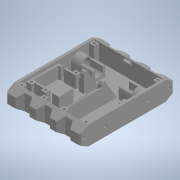
# Autodesk Inventor part: HexBodyV2
Saved by Autodesk Inventor 2020 (Build 240168000, 168)
## iProperties
Created: 2023-12-19
Part Number: HexBodyV2
Material: H TPU
Document SubType Name: Modeling
Designer: smz3rm
Density: 0.941117 g/cm^3
Appearance: Generic(1)
Mass: 179.09 g
Surface Area: 784.016 cm^2
Volume: 190.295 cm^3
BaseThickness: 3.000 mm
TopThickness: 1.778 mm
SideThickness: 4.000 mm
BodyWidth: 118.000 mm
BodyLength: 150.000 mm
BodyHeight: 30.000 mm
DriveMotorHeight: 15.000 mm
WheelWidth: 7.000 mm
WheelGrooveWidth: 5.000 mm
WheelGrooveDia: 18.000 mm
WheelDia: 45.000 mm
WheelPulleyDia: 2.500 mm
M3ScrewInsertBrim: 8.000 mm
M3ScrewDia: 3.100 mm
M3ScrewHeadDia: 6.100 mm
M3ScrewInsertDia: 4.000 mm
M3ScrewInsertDepth: 7.000 mm
DriveMotorOffset: 40.000 mm
DriveMotorHoleDia: 4.200 mm
M3ScrewHeadDepth: 2.200 mm
M3ScrewHeadTaper: -32.50 deg
WheeGuardlSlotWidth: 15.000 mm
WheelGuardScrewOffset: 7.000 mm
FlipperWidth: 20.000 mm
WheelSpokes: 5.000 ul
FlipperRodDia: 2.300 mm
FlipperArmThickness: 4.619 mm
FlipperArmLength: 87.010 mm
FlipperMountOffset: 70.000 mm
FlipperMountThickness: 6.000 mm
FlipperSpikeDrop: 40.009 mm
FlipperSpikeAngle: 30.00 deg
FlipperSpikeWidth: 10.000 mm
WheelGuardSpikeThickness: 8.000 mm
WheelGuardSpikeDrop: 37.700 mm
FlipperArmConnectorLength: 36.000 mm
VM3ScrewInsertDia: 3.750 mm
M2ScrewDia: 2.100 mm
WheelBearingDia: 7.150 mm
TopSupportWidth: 10.000 mm
TopSupportLength: 5.000 mm
ServoToFlipperAxisDistance: 13.685 mm
ServoHeightOffset: 3.000 mm
ServoGearCount: 15.000 ul
ServoGearCenterDistance: 21.290 mm
ServoGearRatio: 1.000 ul
ServoGearWidth: 10.000 mm
ServoToFlipperAxisAngle: 50.00 deg
RidgeCount: 4.000 ul
RidgeSpacing: 32.413 mm
RidgeLength: 20.762 mm
Author: smz3rm
Autodesk Inventor part; units mm, degrees
ref_plane "XZ Plane" through (0, 0, 0) normal (0, 1, 0) x (-1, 0, 0)
ref_plane "XY Plane" through (0, 0, 0) normal (0, 0, 1) x (1, 0, 0)
sketch "Sketch1" plane through (0, 0, 0) normal (1, 0, 0) x (0, 1, 0)
  line L0 (-15, 75) -> (15, 75)
  line L1 (15, 75) -> (15, -75)
  line L2 (15, -75) -> (-15, -75)
  line L3 (-15, -75) -> (-15, 75)
  line L4 (-15, 75) -> (15, -75) construction
  line L5 (15, 75) -> (-15, -75) construction
  line L6 (-21, 0) -> (21, 0) projected
  line L7 (0, -105) -> (0, 105) projected
  line L8 (7.5, -75) -> (-7.5, -75)
  line L9 (-7.5, -75) -> (-15, -62.0096)
  line L10 (-15, -62.0096) -> (-7.5, -49.0192)
  line L11 (-7.5, -49.0192) -> (7.5, -49.0192)
  line L12 (7.5, -49.0192) -> (15, -62.0096)
  line L13 (15, -62.0096) -> (7.5, -75)
  line L14 (-7.5, 75) -> (-15, 62.0096)
  line L15 (15, 62.0096) -> (7.5, 75)
  point P0 (0, 0)
  point P1 (0, -62.0096)
  point P2 (15, -62.0096)
  point P3 (15, 62.0096)
  point P4 (7.5, 75)
  point P5 (-7.5, 75)
  dimension "d0" = 30
  dimension "d1" = 150
  dimension "d25" = 12.9904
  constraints: 28 end point, 4 point on line, 4 symmetric about line, 2 midpoint, 2 parallel, 1 horizontal, 1 perpendicular, 13 other
  measures "d0" distance of L1.end L2.end
  measures "d1" distance of L0.end L1.end
  measures "d25" distance from line of point (0, -62.01) L2
extrude "Extrusion1" add sketch "Sketch1" along normal mid plane 118 contours L0 L7 L6 L3 L14 | L0 L15 L1 L6 L7 | L6 L7 L11 L10 L3 | L6 L1 L12 L11 L7 | L10 L11 L7 L2 L9 | L11 L12 L13 L2 L7
sketch "Sketch2" plane through (-59, 15, 62.4426) normal (0, 1, 0) x (1, 0, 0)
  line L0 (118, 124.4523) -> (118, 0.433) projected
  line L1 (0, 0.433) -> (0, 124.4523) projected
  line L2 (114, 124.4523) -> (4, 124.4523)
  line L3 (4, 124.4523) -> (4, 0.433)
  line L4 (4, 0.433) -> (114, 0.433)
  line L5 (114, 0.433) -> (114, 124.4523)
  line L6 (114, 124.4523) -> (4, 0.433) construction
  line L7 (4, 124.4523) -> (114, 0.433) construction
  line L8 (0, 0.433) -> (118, 0.433) projected
  line L9 (0, 124.4523) -> (118, 124.4523) projected
  line L10 (4, 124.0523) -> (114, 124.0523)
  line L11 (4, 0.833) -> (114, 0.833)
  point P0 (59, 62.4426)
  dimension "d4" = 4
  dimension "d89" = 0.4
  dimension "d90" = 0.4
  constraints: 16 end point, 5 point on line, 3 perpendicular, 2 midpoint, 2 parallel, 1 horizontal
  measures "d4" distance between parallel lines of L1 L3
  measures "d89" distance between parallel lines of L2 L10
  measures "d90" distance between parallel lines of L4 L11
extrude "Extrusion2" cut sketch "Sketch2" against normal blind 27 contours L5 L11 L3 L10
sketch "Sketch3" plane through (-59, -12, 62.4426) normal (0, 1, 0) x (1, 0, 0)
  line L0 (4, 0.833) -> (4, 124.0523) projected
  line L1 (114, 124.0523) -> (114, 0.833) projected
  line L2 (4, 0.833) -> (4, 124.0523) projected
  line L3 (114, 124.0523) -> (114, 0.833) projected
  line L4 (118, 124.4523) -> (118, 0.433) projected
  line L5 (0, 0.433) -> (0, 124.4523) projected
  line L6 (4, 124.0523) -> (12, 124.0523)
  line L7 (12, 124.0523) -> (12, 116.0523)
  line L8 (12, 116.0523) -> (4, 116.0523)
  line L9 (4, 116.0523) -> (4, 124.0523)
  line L10 (-23.6, 62.4426) -> (141.6, 62.4426) projected
  line L11 (59, 167.4426) -> (59, -42.5574) projected
  line L12 (106, 124.0523) -> (106, 116.0523)
  line L13 (106, 116.0523) -> (114, 116.0523)
  line L14 (12, 0.833) -> (12, 8.833)
  line L15 (12, 8.833) -> (4, 8.833)
  line L16 (106, 0.833) -> (106, 8.833)
  line L17 (106, 8.833) -> (114, 8.833)
  line L18 (0, 124.4523) -> (118, 124.4523) projected
  line L19 (0, 0.433) -> (118, 0.433) projected
  line L20 (114, 0.833) -> (4, 0.833) projected
  line L21 (4, 124.0523) -> (114, 124.0523) projected
  line L22 (114, 0.833) -> (4, 0.833) projected
  line L23 (4, 124.0523) -> (114, 124.0523) projected
  line L24 (4, 0.833) -> (4, 124.0523) projected
  line L25 (4, 124.0523) -> (114, 124.0523) projected
  point P0 (59, 62.4426)
  point P1 (4, 8.833)
  point P2 (4, 116.0523)
  point P3 (114, 116.0523)
  point P4 (114, 8.833)
  point P5 (12, 0.833)
  point P6 (106, 0.833)
  point P7 (12, 0.833)
  point P8 (106, 0.833)
  dimension "d8" = 8
  constraints: 20 end point, 9 symmetric about line, 2 horizontal, 2 parallel, 2 perpendicular, 1 collinear, 1 other
  measures "d8" distance of L7.end L8.end
extrude "Extrusion3" add sketch "Sketch3" along normal blind 25.222 contours L0 L15 L14 L20 | L0 L6 L7 L8 | L16 L17 L1 L20 | L13 L12 L21 L1
sketch "Sketch4" plane through (-55, 15, 62.0096) normal (1, 0, 0) x (0, 0, -1)
  circle A0 centre (97.0096, -15) radius 8.25
  line L0 (124.0192, -30) -> (0, -30) projected
  line L1 (137.0096, -7.5) -> (137.0096, -22.5) projected
  circle A1 centre (97.0096, -15) radius 10.25
  line L2 (86.7596, -15) -> (86.7596, -27)
  line L3 (8.4, -27) -> (115.6192, -27) projected
  line L4 (107.2596, -15) -> (107.2596, -27)
  point P0 (62.0096, -15)
  point P1 (0.4, -27)
  dimension "d12" = 16.5
  dimension "d13" = 15
  dimension "d14" = 40
  dimension "d15" = 2
  constraints: 4 end point, 2 centre point, 2 point on circle, 2 point on line, 2 tangent, 2 vertical, 1 coincident
  measures "d12" diameter of A0
  measures "d13" distance from line of L0 A0.centre
  measures "d14" distance from line of L1 A0.centre
  measures "d15" radial gap between concentric circles of A0 A1
extrude "Extrusion4" add sketch "Sketch4" along normal blind 14
sketch "Sketch5" plane through (-41, 15, 62.0096) normal (1, 0, 0) x (0, 0, -1)
  circle A0 centre (97.0096, -15) radius 8.25 projected
  circle A1 centre (97.0096, -15) radius 7.75
  arc A2 (107.2596, -15) -> (86.7596, -15) centre (97.0096, -15) ccw projected
  circle A3 centre (97.0096, -15) radius 8.25 projected
  line L0 (90.9096, -10.2196) -> (87.9426, -10.2196)
  arc A4 (107.2596, -15) -> (86.7596, -15) centre (97.0096, -15) ccw projected
  line L1 (90.9096, -10.2196) -> (90.9096, -27)
  line L2 (107.2596, -27) -> (86.7596, -27) projected
  line L3 (103.1096, -10.2196) -> (106.0766, -10.2196)
  line L4 (103.1096, -10.2196) -> (103.1096, -27)
  line L5 (86.7596, -15) -> (86.7596, -27) projected
  line L6 (107.2596, -27) -> (86.7596, -27) projected
  line L7 (107.2596, -27) -> (107.2596, -15) projected
  point P0 (62.0096, -15)
  point P1 (90.9096, -19.7804)
  point P2 (87.9426, -10.2196)
  point P3 (106.0766, -10.2196)
  point P4 (103.1096, -19.7804)
  dimension "d18" = 15.5
  dimension "d19" = 12.2
  constraints: 8 end point, 4 point on circle, 2 horizontal, 2 point on line, 1 centre point, 1 coincident, 1 parallel, 1 perpendicular
  measures "d18" diameter of A1
  measures "d19" distance between parallel lines of L4 L1
extrude "Extrusion5" add sketch "Sketch5" along normal blind 20 contours A0 L4 A1 L3 | A0 L3 A2 L7 L2 L4 | L4 L2 L1 A0 | A0 L1 A1 L4 | L0 A1 L1 A0 | A0 L1 L2 L5 A2 L0 | A1 L4 | L1 A1
sketch "Sketch6" plane through (-55, 0, -35) normal (1, 0, 0) x (0, 0, -1)
  circle A0 centre (0, 0) radius 2.1
  point P0 (-35, 0)
  dimension "d22" = 4.2
  constraints: 1 centre point
  measures "d22" diameter of A0
extrude "Extrusion6" cut sketch "Sketch6" against normal through all
mirror "Mirror1" about plane through (0, 0, 0) normal (1, 0, 0) of "Extrusion4", "Extrusion5", "Extrusion6"
sketch "Sketch7" plane through (-59, 0, 0) normal (-1, 0, 0) x (0, 0, 1)
  line L0 (-105, 0) -> (105, 0) projected
  circle A0 centre (35, 0) radius 2
  line L1 (75, -7.5) -> (75, 7.5) projected
  point P0 (0, 0)
  dimension "d26" = 4
  dimension "d27" = 40
  constraints: 1 centre point, 1 point on line
  measures "d26" diameter of A0
  measures "d27" distance from line of L1 A0.centre
extrude "Extrusion7" cut sketch "Sketch7" against normal up to surface (4 mm away)
mirror "Mirror2" about plane through (0, 0, 0) normal (1, 0, 0) of "Extrusion7"
sketch "Sketch9" plane through (-59, 0, 0) normal (-1, 0, 0) x (0, 0, 1)
  line L0 (-75, -7.5) -> (-75, 7.5) projected
  line L1 (-75, 0) -> (-62.0096, 0)
  circle A0 centre (-68.5048, 0) radius 2
  line L2 (0, -21) -> (0, 21) projected
  circle A1 centre (68.5048, 0) radius 2
  line L3 (-75, -7.5) -> (-62.0096, -15) projected
  line L4 (-62.0096, -15) -> (-62.0096, 15)
  point P0 (0, 0)
  dimension "d30" = 4
  constraints: 4 end point, 4 midpoint, 2 centre point, 1 symmetric about line, 1 vertical, 1 other
  measures "d30" diameter of A0
extrude "Extrusion8" cut sketch "Sketch9" against normal blind 7 contours A0 L1 | L1 A0 | A1
mirror "Mirror3" about plane through (0, 0, 0) normal (1, 0, 0) of "Extrusion8"
ref_plane "Work Plane1" through (11, 0, 0) normal (1, 0, 0) x (0, 1, 0)
sketch "Sketch10" plane through (11, 0, 0) normal (1, 0, 0) x (0, 1, 0)
  line L0 (-12, 61.6096) -> (-12, -24.75) projected
  line L1 (-12, -1.3627) -> (20.4594, -1.3627)
  line L2 (20.4594, -1.3627) -> (20.4594, -6.8187)
  line L3 (20.4594, -6.8187) -> (-12, -25.5591)
  circle A0 centre (17.3094, -5) radius 1.15
  line L4 (-7.5, -75) -> (7.5, -75) projected
  line L5 (15, -62.0096) -> (15, 62.0096) projected
  line L6 (-12, -24.75) -> (-12, -45.25) projected
  line L7 (-12, -61.6096) -> (-12, 53.6096) projected
  line L8 (20.4594, -6.8187) -> (17.3094, -8.6373)
  line L9 (17.3094, -8.6373) -> (14.1594, -6.8187)
  line L10 (14.1594, -6.8187) -> (14.1594, -3.1813)
  line L11 (14.1594, -3.1813) -> (17.3094, -1.3627)
  line L12 (17.3094, -1.3627) -> (20.4594, -3.1813)
  line L13 (20.4594, -3.1813) -> (20.4594, -6.8187)
  point P0 (0, 0)
  point P1 (18.4594, -5)
  point P2 (15, -9.9706)
  point P3 (15, -1.3627)
  point P4 (-12, -53.6096)
  point P5 (-12, 53.6096)
  dimension "d34" = 2.3
  dimension "d38" = 70
  dimension "d40" = 1.15
  dimension "d41" = 2.3094
  dimension "d44" = 60
  dimension "d45" = 2
  constraints: 18 end point, 4 point on line, 1 coincident, 1 collinear, 1 horizontal, 1 horizontal alignment, 1 perpendicular, 15 other
  measures "d38" distance from line of L4 point (17.309, -5)
  measures "d40" distance of point (17.309, -5) point (18.459, -5)
  measures "d41" distance from line of L5 point (17.309, -5)
  measures "d44" angle of L0 L3
  measures "d45" distance from line of L13 point (18.459, -5)
extrude "Extrusion9" add sketch "Sketch10" along normal blind 6 contours L1 L5 L11 L10 L9 L3 L6 L0 | L1 L11 L5 | L12 L2 L3 L9 L5 L11 | L5 L9 L10 L11 | L5 L9 L3
mirror "Mirror4" about plane through (0, 0, 0) normal (1, 0, 0) of "Extrusion9"
sketch "Sketch12" plane through (-59, -12, 62.4426) normal (0, 1, 0) x (1, 0, 0)
  line L0 (114, 116.0523) -> (114, 107.6926) projected
  line L1 (114, 116.0523) -> (106, 116.0523) projected
  line L2 (106, 116.0523) -> (106, 124.0523) projected
  line L3 (12, 124.0523) -> (12, 116.0523) projected
  line L4 (12, 116.0523) -> (4, 116.0523) projected
  line L5 (4, 107.6926) -> (4, 116.0523) projected
  line L6 (4, 8.833) -> (12, 8.833) projected
  line L7 (12, 8.833) -> (12, 0.833) projected
  line L8 (106, 0.833) -> (106, 8.833) projected
  line L9 (106, 8.833) -> (114, 8.833) projected
  line L10 (47, 0.833) -> (39, 0.833)
  line L11 (39, 0.833) -> (39, 8.833)
  line L12 (39, 8.833) -> (47, 8.833)
  line L13 (47, 8.833) -> (47, 0.833)
  line L14 (59, 167.4426) -> (59, -42.5574) projected
  line L15 (79, 0.833) -> (79, 8.833)
  line L16 (79, 8.833) -> (71, 8.833)
  line L17 (71, 8.833) -> (71, 0.833)
  line L18 (12, 124.0523) -> (106, 124.0523) projected
  line L19 (106, 0.833) -> (12, 0.833) projected
  line L20 (114, 87.1926) -> (80, 87.1926) projected
  line L21 (80, 87.1926) -> (80, 107.6926) projected
  line L22 (80, 107.6926) -> (114, 107.6926) projected
  line L23 (4, 107.6926) -> (38, 107.6926) projected
  line L24 (38, 107.6926) -> (38, 87.1926) projected
  line L25 (38, 87.1926) -> (4, 87.1926) projected
  line L26 (4, 8.833) -> (4, 87.1926) projected
  line L27 (114, 87.1926) -> (114, 8.833) projected
  line L28 (76, 63.8053) -> (70, 63.8053) projected
  line L29 (48, 63.8053) -> (42, 63.8053) projected
  line L30 (70, 63.8053) -> (76, 63.8053) projected
  line L31 (48, 63.8053) -> (42, 63.8053) projected
  line L32 (42, 88.0017) -> (48, 88.0017) projected
  line L33 (48, 88.0017) -> (48, 63.8053) projected
  line L34 (48, 63.8053) -> (42, 63.8053) projected
  line L35 (42, 63.8053) -> (42, 88.0017) projected
  line L36 (76, 88.0017) -> (76, 63.8053) projected
  line L37 (76, 63.8053) -> (70, 63.8053) projected
  line L38 (70, 63.8053) -> (70, 88.0017) projected
  line L39 (70, 88.0017) -> (76, 88.0017) projected
  point P0 (59, 62.4426)
  point P1 (71, 0.833)
  point P2 (79, 0.833)
  dimension "d46" = 8
  dimension "d55" = 12
  constraints: 14 end point, 4 symmetric about line, 2 parallel, 2 perpendicular, 1 collinear, 1 horizontal
  measures "d46" distance of L11.end L12.end
  measures "d55" distance between parallel lines of L14 L13
extrude "Extrusion10" add sketch "Sketch12" along normal blind 25.222 contours L17 L16 L15 L19 | L10 L11 L12 L13
sketch "Sketch13" plane through (-59, 13.222, 62.4426) normal (0, 1, 0) x (1, 0, 0)
  line L0 (12, 116.0523) -> (12, 124.0523) projected
  line L1 (4, 124.0523) -> (12, 124.0523) projected
  line L2 (4, 116.0523) -> (4, 124.0523) projected
  line L3 (4, 116.0523) -> (12, 116.0523) projected
  line L4 (106, 124.0523) -> (114, 124.0523) projected
  line L5 (106, 124.0523) -> (106, 116.0523) projected
  line L6 (106, 116.0523) -> (114, 116.0523) projected
  line L7 (114, 124.0523) -> (114, 116.0523) projected
  line L8 (12, 0.833) -> (4, 0.833) projected
  line L9 (12, 0.833) -> (12, 8.833) projected
  line L10 (12, 8.833) -> (4, 8.833) projected
  line L11 (4, 0.833) -> (4, 8.833) projected
  line L12 (47, 0.833) -> (39, 0.833) projected
  line L13 (47, 0.833) -> (47, 8.833) projected
  line L14 (47, 8.833) -> (39, 8.833) projected
  line L15 (39, 8.833) -> (39, 0.833) projected
  line L16 (114, 8.833) -> (114, 0.833) projected
  line L17 (114, 8.833) -> (106, 8.833) projected
  line L18 (106, 8.833) -> (106, 0.833) projected
  line L19 (114, 0.833) -> (106, 0.833) projected
  line L20 (79, 0.833) -> (79, 8.833) projected
  line L21 (79, 8.833) -> (71, 8.833) projected
  line L22 (71, 8.833) -> (71, 0.833) projected
  line L23 (79, 0.833) -> (71, 0.833) projected
  circle A0 centre (8, 120.0523) radius 1.875
  line L24 (4, 116.0523) -> (4, 124.0523) projected
  line L25 (4, 120.0523) -> (12, 120.0523)
  line L26 (4, 124.0523) -> (12, 124.0523) projected
  line L27 (8, 124.0523) -> (8, 116.0523)
  line L28 (12, 116.0523) -> (4, 116.0523) projected
  line L29 (-23.6, 62.4426) -> (141.6, 62.4426) projected
  line L30 (59, 167.4426) -> (59, -42.5574) projected
  circle A1 centre (110, 120.0523) radius 1.875
  circle A2 centre (8, 4.833) radius 1.875
  circle A3 centre (110, 4.833) radius 1.875
  circle A4 centre (43, 4.833) radius 1.875
  line L31 (39, 0.833) -> (39, 8.833) projected
  line L32 (39, 4.833) -> (47, 4.833)
  line L33 (47, 8.833) -> (39, 8.833) projected
  line L34 (43, 8.833) -> (43, 0.833)
  circle A5 centre (75, 4.833) radius 1.875
  dimension "d91" = 3.75
  dimension "d92" = 3.75
  constraints: 10 midpoint, 8 end point, 6 centre point, 4 symmetric about line, 4 other
  measures "d91" diameter of A0
  measures "d92" diameter of A4
extrude "Extrusion11" cut sketch "Sketch13" against normal blind 7 contours L25 L27 A0 | A0 L27 L25 | A0 L25 L27 | L27 L25 A0 | L34 L32 A4 | A4 L32 L34 | L32 L34 A4 | A4 L34 L32 | A1 | A2 | A3 | A5
sketch "Sketch14" plane through (-59, -12, 62.4426) normal (0, 1, 0) x (1, 0, 0)
  line L0 (7, 63.7574) -> (48, 63.7574)
  line L1 (48, 63.7574) -> (48, 23.7574)
  line L2 (48, 23.7574) -> (7, 23.7574)
  line L3 (7, 23.7574) -> (7, 63.7574)
  line L4 (51, 66.7574) -> (4.5, 66.7574)
  line L5 (4.5, 20.7574) -> (51, 20.7574)
  line L6 (51, 20.7574) -> (51, 66.7574)
  line L7 (40, 66.7574) -> (40, 20.7574)
  line L8 (35, 66.7574) -> (35, 20.7574)
  line L9 (7, 63.7574) -> (35, 63.7574)
  line L10 (4, 43.7574) -> (51, 43.7574)
  line L11 (15.5, 66.7574) -> (15.5, 63.7574)
  line L12 (11, 66.7574) -> (11, 63.7574)
  line L13 (48, 53.7574) -> (54, 53.7574)
  line L14 (54, 53.7574) -> (59, 53.7574)
  line L15 (59, 167.4426) -> (59, -42.5574) projected
  line L16 (48, 68.5926) -> (48, 66.2926) projected
  line L17 (4.5, 66.7574) -> (4, 66.7574)
  line L18 (4, 8.833) -> (4, 87.1926) projected
  line L19 (4, 0.833) -> (4, 124.0523) projected
  line L20 (4.5, 20.7574) -> (4, 20.7574)
  line L21 (35, 23.7574) -> (27, 23.7574)
  line L22 (27, 23.7574) -> (27, 15.7574)
  line L23 (27, 15.7574) -> (35, 15.7574)
  line L24 (35, 15.7574) -> (35, 23.7574)
  line L25 (27, 63.7574) -> (27, 71.7574)
  line L26 (27, 71.7574) -> (35, 71.7574)
  line L27 (35, 71.7574) -> (35, 63.7574)
  line L28 (12, 23.7574) -> (4, 23.7574)
  line L29 (4, 23.7574) -> (4, 15.7574)
  line L30 (4, 15.7574) -> (12, 15.7574)
  line L31 (12, 15.7574) -> (12, 23.7574)
  line L32 (42, 63.8053) -> (42, 88.0017) projected
  line L33 (42, 66.7574) -> (42, 63.7574)
  line L34 (48, 63.7574) -> (48, 63.8053)
  line L35 (48, 63.8053) -> (42, 63.8053) projected
  line L36 (48, 63.7574) -> (48, 63.7574)
  line L37 (48, 63.7574) -> (48, 63.8053)
  point P0 (59, 62.4426)
  point P1 (34.5, 20.5208)
  point P2 (41, 65.8053)
  point P3 (11, 63.7574)
  point P4 (15.5, 63.7574)
  point P5 (48, 67.4426)
  point P6 (48, 43.7574)
  point P7 (40, 23.7574)
  point P8 (27, 66.7574)
  point P9 (35, 66.7574)
  point P10 (35, 20.7574)
  point P11 (27, 20.7574)
  point P12 (12, 20.7574)
  point P13 (40, 63.7574)
  point P14 (42, 63.8053)
  point P15 (42, 63.8053)
  dimension "d57" = 40
  dimension "d58" = 41
  dimension "d60" = 5
  dimension "d134" = 8.5
  dimension "d135" = 4.5
  dimension "d138" = 6
  dimension "d139" = 10
  dimension "d140" = 5
  dimension "d141" = 13.6852
  dimension "d142" = 3
  dimension "d143" = 28
  dimension "d146" = 3
  dimension "d149" = 8
  dimension "d158" = 15
  constraints: 64 end point, 23 point on line, 10 perpendicular, 8 horizontal, 7 parallel, 3 equal length, 3 symmetric about line, 2 collinear, 2 midpoint, 1 vertical, 1 other
  measures "d57" distance of L2.end L0.start
  measures "d58" distance of L1.end L2.end
  measures "d60" distance between parallel lines of L7 L8
  measures "d134" distance between parallel lines of L11 L3
  measures "d135" distance between parallel lines of L11 L12
  measures "d138" distance of L13.start L13.end
  measures "d139" distance between parallel lines of L0 L13
  measures "d140" distance of L14.end L13.end
  measures "d141" vertical distance of L14.end point (48, 67.443)
  measures "d142" distance between parallel lines of L6 L1
  measures "d143" distance between parallel lines of L8 L3
  measures "d146" distance between parallel lines of L0 L4
  measures "d149" distance of L23.end L22.end
  measures "d158" distance between parallel lines of L22 L31
sketch "Sketch20" plane through (55, 15, 61.6096) normal (1, 0, 0) x (0, 0, -1)
  circle A0 centre (26.6096, -15) radius 2 projected
  line L0 (22.6096, -27) -> (30.6096, -27)
  line L1 (30.6096, -27) -> (30.6096, -11)
  line L2 (30.6096, -11) -> (22.6096, -11)
  line L3 (22.6096, -11) -> (22.6096, -27)
  line L4 (8, -27) -> (86.3596, -27) projected
  line L5 (26.6096, -11) -> (26.6096, -15)
  point P0 (61.6096, -15)
  dimension "d96" = 8
  dimension "d97" = 4
  constraints: 10 end point, 2 parallel, 1 horizontal, 1 midpoint, 1 perpendicular, 1 point on line, 1 vertical
  measures "d96" distance of L1.end L2.end
  measures "d97" distance from line of L2 L5.end
extrude "Extrusion17" add sketch "Sketch20" against normal blind 3
sketch "Sketch22" plane through (-17, 20.4594, -6.8187) normal (-1, 0, 0) x (0, 0, 1)
  circle A0 centre (1.8187, -3.15) radius 1.15 projected
  point P0 (6.8187, -20.4594)
extrude "Extrusion19" add sketch "Sketch22" against normal blind 1
mirror "Mirror7" about plane through (0, 0, 0) normal (1, 0, 0) of "Extrusion19"
sketch "Sketch23" plane through (-59, -12, 62.4426) normal (0, 1, 0) x (1, 0, 0)
  line L0 (76, 63.8053) -> (74.4, 63.8053)
  line L1 (74.4, 63.8053) -> (74.4, 8.833)
  line L2 (74.4, 8.833) -> (76, 8.833)
  line L3 (76, 8.833) -> (76, 63.8053)
  line L4 (79, 8.833) -> (71, 8.833) projected
  point P0 (76, 63.8053)
  dimension "d110" = 1.6
  constraints: 8 end point, 2 parallel, 1 coincident, 1 horizontal, 1 perpendicular, 1 point on line
  measures "d110" distance of L2.end L1.end
extrude "Extrusion20" add sketch "Sketch23" along normal up to surface (25.222 mm away)
sketch "Sketch26" plane through (0, 0, 0) normal (1, 0, 0) x (0, 1, 0)
  line L0 (-12, -61.6096) -> (13.222, -61.6096) projected
  line L1 (15, -61.6096) -> (13.222, -61.6096) projected
  line L2 (15, -61.6096) -> (13.222, -61.6096) projected
  line L3 (13.222, -61.6096) -> (-12, -61.6096) projected
  line L4 (13.222, -61.6096) -> (13.222, -56.6096)
  line L5 (13.222, -56.6096) -> (8.222, -61.6096)
  point P0 (0, 0)
  dimension "d121" = 45
  dimension "d122" = 25.222
  dimension "d123" = 5
  constraints: 4 end point, 2 point on line, 1 vertical
  measures "d121" angle of L5 L4
  measures "d122" distance from line of L0.start L4
  measures "d123" distance of L4.start L4.end
extrude "Extrusion22" add sketch "Sketch26" along normal mid plane 10
extrude "Extrusion25" add sketch "Sketch14" along normal blind 22 contours L3 L10 L18 L17 L4 L12 L0 | L3 L28 L18 L10 | L11 L4 L25 L0 | L2 L31 L5 L20 L18 L28 | L25 L4 L8 L0 | L2 L22 L5 L31 | L8 L5 L22 L2 | L25 L26 L27 L4 | L31 L30 L18 L20 L5 | L7 L4 L32 L33 L0 | L2 L1 L10 L6 L5 L7 | L24 L23 L22 L5 | L33 L35 L34 L0
extrude "Extrusion26" add sketch "Sketch14" along normal blind 3 contours L0 L8 L10 L3 | L10 L8 L2 L3 | L10 L7 L2 L8 | L8 L0 L7 L10 | L8 L4 L7 L0 | L2 L7 L5 L8 | L10 L1 L2 L7 | L7 L0 L1 L10 | L7 L4 L32 L33 L0 | L1 L13 L6 L10 | L33 L35 L34 L0 | L1 L34 L35 L32 L4 L6 L13
sketch "Sketch29" plane through (-55, 0, 35) normal (-1, 0, 0) x (0, 0, 1)
  circle A0 centre (0, 0) radius 2 projected
  point P0 (-35, 0)
extrude "Extrusion27" cut sketch "Sketch29" against normal up to surface (3 mm away)
sketch "Sketch30" plane through (-59, 10, 62.4426) normal (0, 1, 0) x (1, 0, 0)
  line L0 (35, 71.7574) -> (27, 71.7574) projected
  line L1 (27, 71.7574) -> (35, 63.7574)
  circle A0 centre (31, 67.7574) radius 1.875
  line L2 (27, 20.7574) -> (27, 15.7574) projected
  line L3 (27, 15.7574) -> (35, 23.7574)
  circle A1 centre (31, 19.7574) radius 1.875
  line L4 (4, 15.7574) -> (12, 15.7574) projected
  line L5 (4, 0.833) -> (4, 124.0523) projected
  line L6 (12, 15.7574) -> (4, 15.7574)
  line L7 (4, 15.7574) -> (4, 23.7574)
  line L8 (4, 23.7574) -> (12, 23.7574)
  line L9 (12, 23.7574) -> (12, 15.7574)
  line L10 (35, 23.7574) -> (7, 23.7574) projected
  line L11 (4, 15.7574) -> (4, 66.7574) projected
  line L12 (4, 23.7574) -> (12, 15.7574)
  circle A2 centre (8, 19.7574) radius 1.875
  line L13 (27, 66.7574) -> (15.5, 66.7574) projected
  line L14 (15.5, 66.7574) -> (15.5, 63.7574) projected
  line L15 (7, 63.7574) -> (11, 63.7574) projected
  line L16 (35, 71.7574) -> (27, 71.7574) projected
  line L17 (27, 71.7574) -> (27, 66.7574) projected
  line L18 (42, 66.7574) -> (42, 63.8053) projected
  line L19 (42, 66.7574) -> (40, 66.7574) projected
  line L20 (40, 66.7574) -> (40, 63.7574) projected
  line L21 (35, 15.7574) -> (35, 23.7574) projected
  line L22 (35, 23.7574) -> (7, 23.7574) projected
  line L23 (7, 23.7574) -> (7, 63.7574) projected
  line L24 (11, 63.7574) -> (11, 66.7574) projected
  line L25 (11, 66.7574) -> (4, 66.7574) projected
  line L26 (4, 15.7574) -> (4, 66.7574) projected
  line L27 (4, 15.7574) -> (12, 15.7574) projected
  line L28 (12, 15.7574) -> (12, 20.7574) projected
  line L29 (12, 20.7574) -> (27, 20.7574) projected
  line L30 (27, 20.7574) -> (27, 15.7574) projected
  line L31 (27, 15.7574) -> (35, 15.7574) projected
  line L32 (15.5, 63.7574) -> (35, 63.7574) projected
  line L33 (42, 63.8053) -> (48, 63.8053) projected
  line L34 (40, 20.7574) -> (51, 20.7574) projected
  line L35 (51, 20.7574) -> (51, 43.7574) projected
  line L36 (51, 43.7574) -> (48, 43.7574) projected
  line L37 (48, 43.7574) -> (48, 23.7574) projected
  line L38 (48, 23.7574) -> (40, 23.7574) projected
  line L39 (40, 23.7574) -> (40, 20.7574) projected
  line L40 (40, 63.7574) -> (48, 63.7574) projected
  line L41 (48, 63.7574) -> (48, 63.8053) projected
  line L42 (35, 63.7574) -> (35, 71.7574) projected
  point P0 (59, 62.4426)
  point P1 (35, 71.7574)
  dimension "d155" = 3.75
  constraints: 14 end point, 3 centre point, 3 midpoint, 2 equal radius, 2 parallel, 1 coincident, 1 collinear, 1 horizontal, 1 perpendicular, 1 point on line
  measures "d155" diameter of A0
extrude "Extrusion28" cut sketch "Sketch30" against normal blind 7 contours A0 L1 | L1 A0 | A1 L3 | L3 A1 | A2 L12 | L12 A2
sketch "Sketch31" plane through (0, 0, 0) normal (0, 0, 1) x (1, 0, 0)
  line L0 (55, -12) -> (55, 4) projected
  line L1 (55, 4) -> (55, -12) projected
  line L2 (55, -12) -> (55, 13.222) projected
  line L3 (55, 15) -> (55, 13.222) projected
  line L4 (55, 15) -> (55, 13.222) projected
  line L5 (55, 13.222) -> (55, -12) projected
  line L6 (55, -12) -> (55, 0) projected
  line L7 (55, 0) -> (55, 0) projected
  line L8 (55, 0) -> (55, -12) projected
  line L9 (55, 13.222) -> (50, 13.222)
  line L10 (50, 13.222) -> (55, 8.222)
  point P0 (0, 0)
  dimension "d160" = 25.222
  dimension "d161" = 5
  dimension "d162" = 45
  constraints: 4 end point, 2 point on line, 1 horizontal
  measures "d160" distance from line of L0.start L9
  measures "d161" distance of L9.start L9.end
  measures "d162" angle of L9 L10
extrude "Extrusion29" add sketch "Sketch31" along normal mid plane 10
sketch "Sketch32" plane through (-55, 15, -61.6096) normal (0, 0, 1) x (1, 0, 0)
  line L0 (102, -27) -> (102, -1.778) projected
  line L1 (8, -1.778) -> (8, -27) projected
  line L2 (0, 0) -> (110, 0) projected
  line L3 (8, -27) -> (102, -27) projected
  line L4 (114, -22.5) -> (-4, -22.5) projected
  line L5 (0, -1.778) -> (8, -1.778) projected
  line L6 (8, -1.778) -> (50, -1.778)
  line L7 (50, -1.778) -> (29, -1.778)
  line L8 (29, -1.778) -> (29, -27)
  line L9 (29, -1.778) -> (41.611, -14.389)
  line L10 (41.611, -14.389) -> (29, -27)
  line L11 (29, -27) -> (16.389, -14.389)
  line L12 (16.389, -14.389) -> (29, -1.778)
  line L13 (55, 6) -> (55, -36) projected
  line L14 (81, -1.778) -> (68.389, -14.389)
  line L15 (68.389, -14.389) -> (81, -27)
  line L16 (81, -27) -> (93.611, -14.389)
  line L17 (93.611, -14.389) -> (81, -1.778)
  point P0 (29, -14.389)
  constraints: 22 end point, 4 symmetric about line, 2 midpoint, 1 horizontal, 1 perpendicular, 1 point on line, 9 other
sketch "Sketch33" plane through (-59, 15, 62.0096) normal (0, 1, 0) x (1, 0, 0)
  line L0 (0, 124.0192) -> (118, 124.0192) projected
  line L1 (118, 137.0096) -> (118, 124.0192) projected
  line L2 (0, 137.0096) -> (118, 137.0096) projected
  line L3 (0, 124.0192) -> (0, 137.0096) projected
  line L4 (0, 124.0192) -> (0, 137.0096) projected
  line L5 (0, 128.0192) -> (59, 128.0192)
  line L6 (0, 124.0192) -> (118, 124.0192) projected
  line L7 (118, 137.0096) -> (0, 137.0096) projected
  line L8 (15.5718, 137.0096) -> (20.7624, 128.0192)
  line L9 (20.7624, 128.0192) -> (15.5718, 119.0289)
  line L10 (15.5718, 119.0289) -> (5.1906, 119.0289)
  line L11 (5.1906, 119.0289) -> (0, 128.0192)
  line L12 (0, 128.0192) -> (5.1906, 137.0096)
  line L13 (5.1906, 137.0096) -> (15.5718, 137.0096)
  line L14 (32.4125, 128.0192) -> (37.6031, 137.0096)
  line L15 (37.6031, 137.0096) -> (47.9843, 137.0096)
  line L16 (47.9843, 137.0096) -> (53.1749, 128.0192)
  line L17 (64.8251, 128.0192) -> (70.0157, 137.0096)
  line L18 (70.0157, 137.0096) -> (80.3969, 137.0096)
  line L19 (80.3969, 137.0096) -> (85.5875, 128.0192)
  line L20 (97.2376, 128.0192) -> (102.4282, 137.0096)
  line L21 (102.4282, 137.0096) -> (112.8094, 137.0096)
  line L22 (112.8094, 137.0096) -> (118, 128.0192)
  line L23 (0, 128.0192) -> (118, 128.0192)
  line L24 (118, 137.0096) -> (118, 124.0192) projected
  point P0 (59, 62.0096)
  point P1 (10.3812, 128.0192)
  point P2 (15.5718, 137.0096)
  point P3 (20.7624, 128.0192)
  point P4 (20.7624, 128.0192)
  point P5 (97.2376, 121.0192)
  point P6 (80.3969, 137.0096)
  point P7 (85.5875, 121.0192)
  point P8 (64.8251, 121.0192)
  point P9 (47.9843, 137.0096)
  point P10 (53.1749, 128.0192)
  dimension "d168" = 4
  dimension "d206" = 32.4125
  constraints: 34 end point, 4 point on line, 1 horizontal, 1 parallel, 1 perpendicular, 34 other
  measures "d168" distance between parallel lines of L0 L5
  measures "d206" distance of L5.start L14.start
extrude "Extrusion30" cut sketch "Sketch33" against normal through all contours L8 L2 L14 L5 | L16 L2 L17 L23 L5 | L23 L19 L2 L20
mirror "Mirror9" about plane through (0, 0, 0) normal (0, 0, 1) of "Extrusion30"
chamfer "Chamfer1" distance 2 angle 45 4 edges at (59, 0, 75) (-59, 0, 75) (-59, 0, -75) (59, 0, -75)
sketch "Sketch39" plane through (-59, 13.222, 62.4426) normal (0, 1, 0) x (1, 0, 0)
  circle A0 centre (8, 120.0523) radius 1.875 projected
  line L0 (4, 116.0523) -> (12, 116.0523) projected
  line L1 (12, 116.0523) -> (12, 124.0523) projected
  line L2 (4, 124.0523) -> (12, 124.0523) projected
  line L3 (4, 116.0523) -> (4, 124.0523) projected
  circle A1 centre (110, 120.0523) radius 1.875 projected
  line L4 (106, 124.0523) -> (106, 116.0523) projected
  line L5 (106, 116.0523) -> (114, 116.0523) projected
  line L6 (114, 124.0523) -> (114, 116.0523) projected
  line L7 (106, 124.0523) -> (114, 124.0523) projected
  circle A2 centre (8, 4.833) radius 1.875 projected
  line L8 (12, 0.833) -> (12, 8.833) projected
  line L9 (12, 8.833) -> (4, 8.833) projected
  line L10 (4, 0.833) -> (4, 8.833) projected
  line L11 (12, 0.833) -> (4, 0.833) projected
  circle A3 centre (43, 4.833) radius 1.875 projected
  line L12 (39, 8.833) -> (39, 0.833) projected
  line L13 (47, 0.833) -> (39, 0.833) projected
  line L14 (47, 0.833) -> (47, 8.833) projected
  line L15 (47, 8.833) -> (39, 8.833) projected
  circle A4 centre (75, 4.833) radius 1.875 projected
  line L16 (79, 0.833) -> (79, 8.833) projected
  line L17 (79, 8.833) -> (76, 8.833) projected
  line L18 (76, 63.8053) -> (76, 8.833) projected
  line L19 (74.4, 63.8053) -> (76, 63.8053) projected
  line L20 (74.4, 8.833) -> (74.4, 63.8053) projected
  line L21 (74.4, 8.833) -> (71, 8.833) projected
  line L22 (71, 8.833) -> (71, 0.833) projected
  line L23 (79, 0.833) -> (71, 0.833) projected
  circle A5 centre (110, 4.833) radius 1.875 projected
  line L24 (114, 0.833) -> (106, 0.833) projected
  line L25 (114, 8.833) -> (114, 0.833) projected
  line L26 (114, 8.833) -> (106, 8.833) projected
  line L27 (106, 8.833) -> (106, 0.833) projected
  line L28 (42, 66.7574) -> (42, 63.8053) projected
  line L29 (42, 65.624) -> (42, 63.8053) projected
  line L30 (42, 69.2613) -> (42, 65.624) projected
  line L31 (42, 88.0017) -> (42, 69.2613) projected
  line L32 (42, 66.7574) -> (42, 88.0017) projected
  line L33 (48, 88.0017) -> (48, 69.2613) projected
  line L34 (42, 88.0017) -> (48, 88.0017) projected
  line L35 (42, 88.0017) -> (42, 69.2613) projected
  line L36 (48, 69.2613) -> (42, 69.2613) projected
  line L37 (48, 68.5926) -> (48, 66.2926) projected
  line L38 (48, 63.7574) -> (48, 66.7574) projected
  line L39 (48, 88.0017) -> (48, 66.7574) projected
  line L40 (48, 88.0017) -> (48, 69.2613) projected
  line L41 (48, 69.2613) -> (48, 65.624) projected
  line L42 (48, 65.624) -> (48, 63.8053) projected
  line L43 (48, 63.7574) -> (48, 63.8053) projected
  line L44 (42, 63.8053) -> (48, 63.8053) projected
  line L45 (48, 63.8053) -> (42, 63.8053) projected
  line L46 (48, 88.0017) -> (48, 69.2613) projected
  line L47 (42, 88.0017) -> (42, 69.2613) projected
  line L48 (70, 88.0017) -> (70, 69.2613) projected
  line L49 (70, 69.2613) -> (76, 69.2613) projected
  line L50 (76, 88.0017) -> (76, 69.2613) projected
  line L51 (70, 88.0017) -> (76, 88.0017) projected
  line L52 (70, 88.0017) -> (70, 69.2613) projected
  line L53 (70, 63.8053) -> (70, 88.0017) projected
  line L54 (70, 65.624) -> (70, 63.8053) projected
  line L55 (70, 69.2613) -> (70, 65.624) projected
  line L56 (70, 68.5926) -> (70, 66.2926) projected
  line L57 (74.4, 63.8053) -> (76, 63.8053) projected
  line L58 (70, 63.8053) -> (76, 63.8053) projected
  line L59 (74.4, 63.8053) -> (70, 63.8053) projected
  line L60 (76, 88.0017) -> (76, 69.2613) projected
  line L61 (76, 69.2613) -> (76, 65.624) projected
  line L62 (76, 65.624) -> (76, 63.8053) projected
  line L63 (76, 63.8053) -> (76, 8.833) projected
  line L64 (76, 88.0017) -> (76, 8.833) projected
  line L65 (12, 116.0523) -> (12, 124.0523) projected
  line L66 (12, 124.0523) -> (106, 124.0523)
  line L67 (4, 124.0523) -> (114, 124.0523) projected
  line L68 (4, 0.833) -> (4, 8.833) projected
  line L69 (4, 124.0523) -> (4, 0.833)
  line L70 (4, 0.833) -> (47, 0.833)
  line L71 (114, 0.833) -> (4, 0.833) projected
  line L72 (42, 63.8053) -> (48, 63.8053) projected
  line L73 (106, 116.0523) -> (114, 116.0523) projected
  line L74 (114, 8.833) -> (114, 0.833) projected
  line L75 (114, 116.0523) -> (114, 8.833)
  line L76 (106, 0.833) -> (79, 0.833)
  line L77 (0, -2.6466) -> (0, 127.5318) projected
  line L78 (0, 127.5318) -> (118, 127.5318) projected
  line L79 (118, 127.5318) -> (118, -2.6466) projected
  line L80 (118, -2.6466) -> (0, -2.6466) projected
  line L81 (48, 73.4398) -> (48, 63.8053) projected
  line L82 (48, 63.8053) -> (42, 63.8053) projected
  line L83 (42, 63.8053) -> (42, 73.4398) projected
  line L84 (42, 73.4398) -> (48, 73.4398) projected
  circle A6 centre (8, 4.833) radius 1.875 projected
  circle A7 centre (110, 4.833) radius 1.875 projected
  circle A8 centre (110, 120.0523) radius 1.875 projected
  circle A9 centre (43, 4.833) radius 1.875 projected
  circle A10 centre (75, 4.833) radius 1.875 projected
  circle A11 centre (8, 120.0523) radius 1.875 projected
  line L85 (12, 124.0523) -> (12, 116.0523) projected
  line L86 (12, 116.0523) -> (4, 116.0523) projected
  line L87 (4, 116.0523) -> (4, 8.833) projected
  line L88 (4, 8.833) -> (4, 0.833) projected
  line L89 (4, 0.833) -> (12, 0.833) projected
  line L90 (12, 0.833) -> (39, 0.833) projected
  line L91 (39, 0.833) -> (39, 8.833) projected
  line L92 (39, 8.833) -> (47, 8.833) projected
  line L93 (47, 8.833) -> (47, 0.833) projected
  line L94 (47, 0.833) -> (71, 0.833) projected
  line L95 (71, 0.833) -> (71, 8.833) projected
  line L96 (71, 8.833) -> (74.4, 8.833) projected
  line L97 (74.4, 8.833) -> (74.4, 63.8053) projected
  line L98 (76, 63.8053) -> (74.4, 63.8053) projected
  line L99 (76, 73.4398) -> (76, 63.8053) projected
  line L100 (70, 73.4398) -> (76, 73.4398) projected
  line L101 (70, 63.8053) -> (70, 73.4398) projected
  line L102 (74.4, 63.8053) -> (70, 63.8053) projected
  line L103 (12, 124.0523) -> (4, 124.0523) projected
  line L104 (54, 124.0523) -> (12, 124.0523) projected
  line L105 (54, 119.0523) -> (54, 124.0523) projected
  line L106 (64, 119.0523) -> (54, 119.0523) projected
  line L107 (64, 124.0523) -> (64, 119.0523) projected
  line L108 (106, 124.0523) -> (64, 124.0523) projected
  line L109 (106, 116.0523) -> (106, 124.0523) projected
  line L110 (114, 116.0523) -> (106, 116.0523) projected
  line L111 (114, 67.4426) -> (114, 116.0523) projected
  line L112 (109, 67.4426) -> (114, 67.4426) projected
  line L113 (109, 57.4426) -> (109, 67.4426) projected
  line L114 (114, 57.4426) -> (109, 57.4426) projected
  line L115 (114, 8.833) -> (114, 57.4426) projected
  line L116 (106, 8.833) -> (114, 8.833) projected
  line L117 (106, 0.833) -> (106, 8.833) projected
  line L118 (79, 0.833) -> (106, 0.833) projected
  line L119 (71, 0.833) -> (79, 0.833) projected
  line L120 (4, 124.0523) -> (4, 116.0523) projected
  line L121 (4, 8.833) -> (12, 8.833) projected
  line L122 (12, 8.833) -> (12, 0.833) projected
  line L123 (39, 0.833) -> (47, 0.833) projected
  line L124 (76, 63.8053) -> (76, 8.833) projected
  line L125 (76, 8.833) -> (79, 8.833) projected
  line L126 (79, 8.833) -> (79, 0.833) projected
  line L127 (64, 124.0523) -> (54, 124.0523) projected
  line L128 (114, 124.0523) -> (106, 124.0523) projected
  line L129 (114, 116.0523) -> (114, 124.0523) projected
  line L130 (114, 57.4426) -> (114, 67.4426) projected
  line L131 (114, 0.833) -> (114, 8.833) projected
  line L132 (106, 0.833) -> (114, 0.833) projected
  line L133 (48, 73.4398) -> (70, 73.4398)
  line L134 (70, 88.0017) -> (70, 69.2613) projected
  line L135 (52.5, 73.4398) -> (52.5, 82.0878)
  line L136 (59, 73.4398) -> (59, 82.0878)
  line L137 (65.5, 73.4398) -> (65.5, 82.0878)
  line L138 (52.5, 82.0878) -> (65.5, 82.0878)
  line L139 (0, -2.6466) -> (0, 127.5318) projected
  line L140 (0, 127.5318) -> (118, 127.5318) projected
  line L141 (118, 127.5318) -> (118, -2.6466) projected
  line L142 (118, -2.6466) -> (0, -2.6466) projected
  line L143 (48, 73.4398) -> (48, 63.8053) projected
  line L144 (48, 63.8053) -> (42, 63.8053) projected
  line L145 (42, 63.8053) -> (42, 73.4398) projected
  line L146 (42, 73.4398) -> (48, 73.4398) projected
  circle A12 centre (8, 4.833) radius 1.875 projected
  circle A13 centre (110, 4.833) radius 1.875 projected
  circle A14 centre (110, 120.0523) radius 1.875 projected
  circle A15 centre (43, 4.833) radius 1.875 projected
  circle A16 centre (75, 4.833) radius 1.875 projected
  circle A17 centre (8, 120.0523) radius 1.875 projected
  line L147 (12, 124.0523) -> (12, 116.0523) projected
  line L148 (12, 116.0523) -> (4, 116.0523) projected
  line L149 (4, 116.0523) -> (4, 8.833) projected
  line L150 (4, 8.833) -> (4, 0.833) projected
  line L151 (4, 0.833) -> (12, 0.833) projected
  line L152 (12, 0.833) -> (39, 0.833) projected
  line L153 (39, 0.833) -> (39, 8.833) projected
  line L154 (39, 8.833) -> (47, 8.833) projected
  line L155 (47, 8.833) -> (47, 0.833) projected
  line L156 (47, 0.833) -> (71, 0.833) projected
  line L157 (71, 0.833) -> (71, 8.833) projected
  line L158 (71, 8.833) -> (74.4, 8.833) projected
  line L159 (74.4, 8.833) -> (74.4, 63.8053) projected
  line L160 (76, 63.8053) -> (74.4, 63.8053) projected
  line L161 (76, 73.4398) -> (76, 63.8053) projected
  line L162 (70, 73.4398) -> (76, 73.4398) projected
  line L163 (70, 63.8053) -> (70, 73.4398) projected
  line L164 (74.4, 63.8053) -> (70, 63.8053) projected
  line L165 (12, 124.0523) -> (4, 124.0523) projected
  line L166 (54, 124.0523) -> (12, 124.0523) projected
  line L167 (54, 119.0523) -> (54, 124.0523) projected
  line L168 (64, 119.0523) -> (54, 119.0523) projected
  line L169 (64, 124.0523) -> (64, 119.0523) projected
  line L170 (106, 124.0523) -> (64, 124.0523) projected
  line L171 (106, 116.0523) -> (106, 124.0523) projected
  line L172 (114, 116.0523) -> (106, 116.0523) projected
  line L173 (114, 67.4426) -> (114, 116.0523) projected
  line L174 (109, 67.4426) -> (114, 67.4426) projected
  line L175 (109, 57.4426) -> (109, 67.4426) projected
  line L176 (114, 57.4426) -> (109, 57.4426) projected
  line L177 (114, 8.833) -> (114, 57.4426) projected
  line L178 (106, 8.833) -> (114, 8.833) projected
  line L179 (106, 0.833) -> (106, 8.833) projected
  line L180 (79, 0.833) -> (106, 0.833) projected
  line L181 (71, 0.833) -> (79, 0.833) projected
  line L182 (4, 124.0523) -> (4, 116.0523) projected
  line L183 (4, 8.833) -> (12, 8.833) projected
  line L184 (12, 8.833) -> (12, 0.833) projected
  line L185 (39, 0.833) -> (47, 0.833) projected
  line L186 (76, 63.8053) -> (76, 8.833) projected
  line L187 (76, 8.833) -> (79, 8.833) projected
  line L188 (79, 8.833) -> (79, 0.833) projected
  line L189 (64, 124.0523) -> (54, 124.0523) projected
  line L190 (114, 124.0523) -> (106, 124.0523) projected
  line L191 (114, 116.0523) -> (114, 124.0523) projected
  line L192 (114, 57.4426) -> (114, 67.4426) projected
  line L193 (114, 0.833) -> (114, 8.833) projected
  line L194 (106, 0.833) -> (114, 0.833) projected
  line L195 (70, 68.5926) -> (70, 66.2926) projected
  line L196 (70, 67.4426) -> (48, 67.4426)
  line L197 (48, 68.5926) -> (48, 66.2926) projected
  line L198 (47, 0.833) -> (47, 8.833) projected
  line L199 (47, 8.833) -> (47, 63.8053)
  line L200 (71, 8.833) -> (71, 63.8053)
  point P0 (59, 62.4426)
  dimension "d211" = 13
  dimension "d213" = 14.6452
  constraints: 26 end point, 5 collinear, 4 midpoint, 2 perpendicular, 2 point on line, 2 symmetric about line, 2 vertical, 1 horizontal, 1 parallel, 10 other
  measures "d211" distance of L135.end L137.end
  measures "d213" distance between parallel lines of L196 L138
equation "\"d0\" = BodyHeight"
equation "\"d1\" = BodyLength"
equation "\"d2\" = BodyWidth"
equation "\"d4\" = SideThickness"
equation "\"d5\" = BodyHeight - BaseThickness"
equation "\"d8\" = M3ScrewInsertBrim"
equation "\"d10\" = -BaseThickness + BodyHeight - TopThickness"
equation "\"d13\" = DriveMotorHeight"
equation "\"d14\" = DriveMotorOffset"
equation "\"d22\" = DriveMotorHoleDia"
equation "\"d26\" = M3ScrewInsertDia"
equation "\"d27\" = DriveMotorOffset"
equation "\"d30\" = M3ScrewInsertDia"
equation "\"d31\" = M3ScrewInsertDepth"
equation "\"d38\" = FlipperMountOffset"
equation "\"d40\" = 0.5 * d34"
equation "\"d41\" = 0.5 * FlipperArmThickness"
equation "\"d42\" = FlipperMountThickness"
equation "\"d46\" = M3ScrewInsertBrim"
equation "\"d48\" = -BaseThickness + BodyHeight - TopThickness"
equation "\"d53\" = M3ScrewInsertDepth"
equation "\"BaseThickness\" = 3"
equation "\"TopThickness\" = 1.778"
equation "\"SideThickness\" = 4"
equation "\"BodyWidth\" = 118"
equation "\"BodyLength\" = 150"
equation "\"BodyHeight\" = 30"
equation "\"DriveMotorHeight\" = 0.5 * BodyHeight"
equation "\"WheelDia\" = 45"
equation "\"WheelWidth\" = 7"
equation "\"WheelGrooveWidth\" = 5"
equation "\"WheelGrooveDia\" = 0.4 * WheelDia"
equation "\"WheelPulleyDia\" = 2.5"
equation "\"M3ScrewInsertBrim\" = 8"
equation "\"M3ScrewDia\" = 3.1"
equation "\"M3ScrewHeadDia\" = 6.1"
equation "\"M3ScrewInsertDia\" = 4"
equation "\"M3ScrewInsertDepth\" = 7"
equation "\"DriveMotorOffset\" = 40"
equation "\"DriveMotorHoleDia\" = 4.2"
equation "\"M3ScrewHeadDepth\" = 2.2"
equation "\"M3ScrewHeadTaper\" = -32.5deg"
equation "\"WheelGuardScrewOffset\" = 7"
equation "\"FlipperArmLength\" = 2.5 * M3ScrewInsertBrim - FlipperMountOffset + BodyLength - 0.433013 * BodyHeight"
equation "\"FlipperWidth\" = 20"
equation "\"WheelSpokes\" = 5"
equation "\"FlipperRodDia\" = 2.3"
equation "\"FlipperMountOffset\" = 70"
equation "\"FlipperMountThickness\" = 6"
equation "\"FlipperSpikeWidth\" = 10"
equation "\"FlipperSpikeAngle\" = 30deg"
equation "\"WheelGuardSpikeThickness\" = 8"
equation "\"ServoToFlipperAxisDistance\" = 13.68521"
equation "\"FlipperArmConnectorLength\" = 36"
equation "\"VM3ScrewInsertDia\" = 3.75"
equation "\"M2ScrewDia\" = 2.1"
equation "\"WheelBearingDia\" = 7.15"
equation "\"TopSupportWidth\" = 10"
equation "\"TopSupportLength\" = 5"
equation "\"ServoHeightOffset\" = 3"
equation "\"ServoGearCount\" = 15"
equation "\"ServoGearCenterDistance\" = 21.29041"
equation "\"ServoGearRatio\" = 1"
equation "\"ServoGearWidth\" = 10"
equation "\"ServoToFlipperAxisAngle\" = 50deg"
equation "\"RidgeCount\" = 4"
equation "\"RidgeSpacing\" = 32.41253"
equation "\"RidgeLength\" = 20.7624"
equation "\"FlipperArmThickness\" = 4.618802"
body "Solid1"
